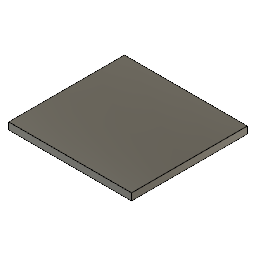
top-plate v1 (Autodesk Fusion 360 design; units mm, degrees)
Autodesk Fusion 360 part; units mm, degrees
sketch "Sketch1" plane through (0, 0, 0) normal (0, 0, 1) x (1, 0, 0)
  line L0 (0, 0) -> (76, 0)
  line L1 (76, 0) -> (76, 76)
  line L2 (76, 76) -> (0, 76)
  line L3 (0, 76) -> (0, 0)
  dimension "d1" = 76
  dimension "d2" = 76
  constraint horizontal L0
  constraint vertical L1
  constraint horizontal L2
  constraint vertical L3
  constraint coincident L0.start L3.end
  measures "d1" distance of L0.start L0.end
  measures "d2" distance of L0.start L2.end
sketch "Sketch2" plane through (0, 0, 6.35) normal (0, 0, 1) x (-1, 0, 0)
  line L0 (0, -76) -> (0, 0)
  line L1 (0, 0) -> (-76, 0)
  line L2 (-76, 0) -> (-76, -76)
  line L3 (-76, -76) -> (0, -76)
  line L4 (-52, -66) -> (-38, -66)
  line L5 (-38, -66) -> (-38, -91)
  line L6 (-38, -91) -> (-52, -91)
  line L7 (-52, -91) -> (-52, -66)
  dimension "d5" = 14
  dimension "d6" = 25
  dimension "d7" = 24
  dimension "d8" = 10
  constraint horizontal L4
  constraint vertical L5
  constraint horizontal L6
  constraint vertical L7
  measures "d5" distance of L4.start L4.end
  measures "d6" distance of L4.start L6.end
  measures "d7" distance of L2 L7
  measures "d8" distance of L3 L4
sketch "Sketch3" plane through (0, 0, 16.35) normal (0, 0, 1) x (-1, 0, 0)
  line L0 (-52, -86) -> (-38, -86)
  line L1 (-38, -86) -> (-38, -76)
  line L2 (-38, -76) -> (-52, -76)
  line L3 (-52, -76) -> (-52, -86)
  line L4 (-50, -80) -> (-40, -80)
  line L5 (-40, -80) -> (-40, -95)
  line L6 (-40, -95) -> (-50, -95)
  line L7 (-50, -95) -> (-50, -80)
  constraint horizontal L4
  constraint vertical L5
  constraint horizontal L6
  constraint vertical L7
sketch "Sketch4" plane through (40, 0, 0) normal (1, 0, 0) x (0, 1, 0)
  line L0 (80, 6.35) -> (86, 6.35)
  arc A0 (86, 6.35) -> (86, 16.35) centre (86, 11.35) ccw
  line L1 (86, 16.35) -> (80, 16.35)
  line L2 (80, 16.35) -> (80, 6.35)
  circle A1 centre (86, 11.35) radius 3.25
  dimension "d17" = 6.5
  constraint concentric A0 A1
  measures "d17" diameter of A1
sketch "Sketch5" plane through (0, 0, 6.35) normal (0, 0, 1) x (-1, 0, 0)
  line L0 (5, 0) -> (5, 5)
  line L1 (-81, -76) -> (-76.6575, -76)
  line L2 (-76.6575, -76) -> (-76.6575, -71)
  line L3 (-76.6575, -71) -> (-81, -71)
  line L4 (-81, -71) -> (-81, -76)
  line L5 (-76, -76) -> (-81, -76)
  line L6 (-81, -76) -> (-81, -71)
  line L7 (-81, -71) -> (-76, -71)
  line L8 (-76, -71) -> (-76, -76)
  line L9 (-76, 5) -> (-81, 5)
  line L10 (-81, 5) -> (-81, 0)
  line L11 (-81, 0) -> (-76, 0)
  line L12 (-76, 0) -> (-76, 5)
  line L13 (-81, 5) -> (-76, 5)
  line L14 (-76, 5) -> (-76, 0)
  line L15 (-76, 0) -> (-81, 0)
  line L16 (-81, 0) -> (-81, 5)
  line L17 (0, 5) -> (0, 0)
  line L18 (5, 5) -> (0, 5)
  line L19 (0, 0) -> (5, 0)
  dimension "d26" = 5
  dimension "d27" = 5
  dimension "d28" = 5
  dimension "d29" = 5
  dimension "d30" = 5
  dimension "d31" = 5
  dimension "d32" = 5
  constraint horizontal L1
  constraint vertical L2
  constraint horizontal L3
  constraint vertical L4
  constraint horizontal L5
  constraint vertical L6
  constraint horizontal L7
  constraint vertical L8
  constraint horizontal L9
  constraint vertical L10
  constraint horizontal L11
  constraint vertical L12
  constraint horizontal L13
  constraint vertical L14
  constraint horizontal L15
  constraint vertical L16
  measures "d26" distance of L1.start L3.end
  measures "d27" distance of L5.start L1.start
  measures "d28" distance of L5.start L7.end
  measures "d29" distance of L9.start L9.end
  measures "d30" distance of L9.start L11.end
  measures "d31" distance of L9.end L9.start
  measures "d32" distance of L9.end L10.end
ref_plane "WorkPlane1" through (78.5, -2.5, 31.35) normal (0, 0, 1) x (1, 0, 0)
sketch "Sketch6" plane through (-2.5, -2.5, 31.35) normal (0, 0, 1) x (1, 0, 0)
  line L0 (-2.5, 78.5) -> (83.5, 78.5)
  line L1 (83.5, 78.5) -> (83.5, -2.5)
  line L2 (83.5, -2.5) -> (-2.5, -2.5)
  line L3 (-2.5, -2.5) -> (-2.5, 78.5)
  point P0 (83.5, -2.5)
  point P1 (78.5, 78.5)
  constraint horizontal L0
  constraint vertical L1
  constraint horizontal L2
  constraint vertical L3
  constraint coincident P0 L1.end
extrude "Extrude1" add sketch "Sketch6" along normal blind 5 in component "Component"
move_body "Move1" bodies 1 to x (1, 0, 0) y (0, 1, 0) z (0, 0, 1) at (0, 0, 5) in component "Component"
component "Component" placed x (1, 0, 0) y (0, 1, 0) z (0, 0, 1) at (0, 0, 0)
